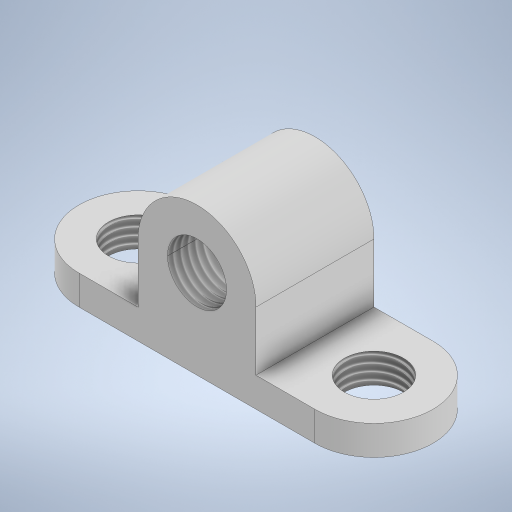
# Autodesk Inventor part: Tarea#1 Adrian Montalvan
Saved by Autodesk Inventor 2024 (Build 280153000, 153)
## iProperties
Created: 2024-01-27
Part Number: Tarea#1 Adrian Montalvan
Material: Genérico
Document SubType Name: Modeling
Designer: Adrian Montalvan
Density: 1 g/cm^3
Appearance: Valor por defecto
Author: Adrian Montalvan
Autodesk Inventor part; units mm, degrees
ref_plane "YZ Plane" through (0, 0, 0) normal (1, 0, 0) x (0, 1, 0)
ref_plane "XZ Plane" through (0, 0, 0) normal (0, 1, 0) x (-1, 0, 0)
ref_plane "XY Plane" through (0, 0, 0) normal (0, 0, 1) x (1, 0, 0)
sketch "Boceto1" plane through (0, 0, 0) normal (0, 0, 1) x (1, 0, 0)
  line L0 (-20, -15) -> (20, -15)
  line L1 (20, -15) -> (20, 15)
  line L2 (20, 15) -> (-20, 15)
  line L3 (-20, 15) -> (-20, -15)
  line L4 (-20, -15) -> (20, 15) construction
  line L5 (20, -15) -> (-20, 15) construction
  point P0 (0, 0)
  dimension "d0" = 40
  dimension "d1" = 30
  constraints: 12 end point, 2 midpoint, 2 parallel, 1 horizontal, 1 perpendicular
  measures "d0" distance of L2.end L1.end
  measures "d1" distance of L1.end L0.end
extrude "Extrusión1" add sketch "Boceto1" along normal blind 40
sketch "Boceto2" plane through (0, 0, 40) normal (0, 0, 1) x (1, 0, 0)
  line L0 (20, 15) -> (-20, 15) projected
  circle A0 centre (0, 15) radius 10
  circle A1 centre (0, 15) radius 20
  point P0 (0, 0)
  point P1 (-10, 15)
  point P2 (10, 15)
  dimension "d4" = 20
  constraints: 1 centre point, 1 coincident, 1 midpoint, 3 other
  measures "d4" diameter of A0
extrude "Extrusión2" add sketch "Boceto2" against normal blind 40 contours L0 A0 A1 picked at (-3.5694, 31.1605)
sketch "Boceto3" plane through (0, 0, 40) normal (0, 0, 1) x (1, 0, 0)
  circle A0 centre (0, 15.0754) radius 10
  point P0 (0, 0)
  dimension "d7" = 20
  constraints: 1 centre point
  measures "d7" diameter of A0
extrude "Extrusión3" cut sketch "Boceto3" against normal blind 40
sketch "Boceto4" plane through (20, -15, 40) normal (1, 0, 0) x (0, 0, -1)
  line L0 (40, 30) -> (40, 0) projected
  line L1 (40, 0) -> (0, 0)
  line L2 (0, 0) -> (0, 10)
  line L3 (0, 10) -> (40, 10)
  line L4 (40, 10) -> (40, 0)
  point P0 (40, 15)
  dimension "d10" = 40
  dimension "d11" = 10
  constraints: 8 end point, 2 parallel, 1 horizontal, 1 perpendicular
  measures "d10" distance of L2.end L3.end
  measures "d11" distance of L1.end L2.end
extrude "Extrusión4" add sketch "Boceto4" along normal blind 20
sketch "Boceto5" plane through (20, -5, 40) normal (0, 1, 0) x (1, 0, 0)
  line L0 (20, 40) -> (20, 0) projected
  circle A0 centre (20, 20) radius 10
  circle A1 centre (20, 20) radius 20
  point P0 (-20, 40)
  point P1 (20, 30)
  point P2 (20, 10)
  dimension "d14" = 20
  constraints: 1 centre point, 1 coincident, 1 midpoint, 3 other
  measures "d14" diameter of A0
extrude "Extrusión5" add sketch "Boceto5" against normal blind 10 contours A1 L0 A0 picked at (36.4159, 17.7748)
sketch "Boceto6" plane through (20, -5, 40) normal (0, 1, 0) x (1, 0, 0)
  line L0 (20, 10) -> (20, 30) projected
  circle A0 centre (20, 20) radius 10
  point P0 (-20, 40)
  dimension "d17" = 20
  constraints: 1 centre point, 1 midpoint
  measures "d17" diameter of A0
extrude "Extrusión6" cut sketch "Boceto6" against normal blind 10 contours A0 L0 picked at (18.4509, 17.0485)
sketch "Boceto7" plane through (-20, -15, 0) normal (-1, 0, 0) x (0, 0, 1)
  point P0 (0, 15)
sketch "Boceto8" plane through (-20, -15, 0) normal (-1, 0, 0) x (0, 0, 1)
  line L0 (0, 0) -> (40, 0) projected
  line L1 (0, 0) -> (40, 0)
  line L2 (40, 0) -> (40, 10)
  line L3 (40, 10) -> (0, 10)
  line L4 (0, 10) -> (0, 0)
  point P0 (0, 15)
  dimension "d20" = 40
  dimension "d21" = 10
  constraints: 8 end point, 2 parallel, 1 horizontal, 1 perpendicular
  measures "d20" distance of L3.end L2.end
  measures "d21" distance of L2.end L1.end
extrude "Extrusión7" add sketch "Boceto8" along normal blind 20
sketch "Boceto9" plane through (-20, -5, 40) normal (0, 1, 0) x (1, 0, 0)
  line L0 (-20, 40) -> (-20, 0) projected
  circle A0 centre (-20, 20) radius 10
  circle A1 centre (-20, 20) radius 20
  point P0 (20, 40)
  point P1 (-20, 10)
  point P2 (-20, 30)
  dimension "d24" = 20
  dimension "d25" = 40
  constraints: 2 centre point, 1 coincident, 1 midpoint
  measures "d24" diameter of A0
  measures "d25" diameter of A1
extrude "Extrusión8" add sketch "Boceto9" against normal blind 10 contours L0 A0 A1 picked at (-22.3932, 3.6239)
sketch "Boceto10" plane through (-20, -5, 40) normal (0, 1, 0) x (1, 0, 0)
  line L0 (-20, 30) -> (-20, 10) projected
  circle A0 centre (-20, 20) radius 10
  point P0 (20, 40)
  dimension "d28" = 20
  constraints: 1 centre point, 1 midpoint
  measures "d28" diameter of A0
extrude "Extrusión9" cut sketch "Boceto10" against normal blind 10 contours A0 L0 picked at (-17.3939, 17.9217)
thread "Rosca1" size "M20x2.5" class "6H" standard "ANSI Metric M Profile" full length
thread "Rosca2" size "M20x2.5" class "6H" standard "ANSI Metric M Profile" full length
thread "Rosca3" size "M20x2.5" class "6H" standard "ANSI Metric M Profile" full length
thread "Rosca4" size "M20x2.5" class "6H" standard "ANSI Metric M Profile" full length
